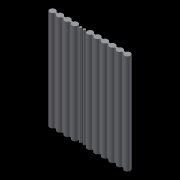
# Autodesk Inventor part: 3d_LM-Welding_Tooling - Wire Jacket
Saved by Autodesk Inventor 2018.3 (Build 223284000, 284)
## iProperties
Created: 2026-01-21
Part Number: 3d_LM-Welding_Tooling - Wire Jacket
Material: Genérico
Document SubType Name: Modeling
Designer: aca6
Density: 1 g/cm^3
Appearance: Valor por defecto
Author: aca6
Autodesk Inventor part; units mm, degrees
ref_plane "YZ Plane" through (0, 0, 0) normal (1, 0, 0) x (0, 1, 0)
ref_plane "XZ Plane" through (0, 0, 0) normal (0, 1, 0) x (-1, 0, 0)
ref_plane "XY Plane" through (0, 0, 0) normal (0, 0, 1) x (1, 0, 0)
sketch "Sketch1" plane through (0, 0, 0) normal (0, 0, 1) x (1, 0, 0)
  line L0 (25, -2) -> (24.25, -2) projected
  line L1 (25, 2) -> (25, -2) projected
  line L2 (24.25, 2) -> (25, 2) projected
  arc A0 (20.8229, 1.5) -> (24.25, 2) centre (22.5, 2) ccw projected
  line L3 (19.6771, 1.5) -> (20.8229, 1.5) projected
  arc A1 (16.3229, 1.5) -> (19.6771, 1.5) centre (18, 2) ccw projected
  line L4 (15.1771, 1.5) -> (16.3229, 1.5) projected
  arc A2 (11.8229, 1.5) -> (15.1771, 1.5) centre (13.5, 2) ccw projected
  line L5 (10.6771, 1.5) -> (11.8229, 1.5) projected
  arc A3 (7.3229, 1.5) -> (10.6771, 1.5) centre (9, 2) ccw projected
  line L6 (6.1771, 1.5) -> (7.3229, 1.5) projected
  arc A4 (2.8229, 1.5) -> (6.1771, 1.5) centre (4.5, 2) ccw projected
  line L7 (1.6771, 1.5) -> (2.8229, 1.5) projected
  arc A5 (-1.6771, 1.5) -> (1.6771, 1.5) centre (0, 2) ccw projected
  line L8 (-2.8229, 1.5) -> (-1.6771, 1.5) projected
  arc A6 (-6.1771, 1.5) -> (-2.8229, 1.5) centre (-4.5, 2) ccw projected
  line L9 (-7.3229, 1.5) -> (-6.1771, 1.5) projected
  arc A7 (-10.6771, 1.5) -> (-7.3229, 1.5) centre (-9, 2) ccw projected
  line L10 (-11.8229, 1.5) -> (-10.6771, 1.5) projected
  arc A8 (-15.1771, 1.5) -> (-11.8229, 1.5) centre (-13.5, 2) ccw projected
  line L11 (-16.3229, 1.5) -> (-15.1771, 1.5) projected
  arc A9 (-19.6771, 1.5) -> (-16.3229, 1.5) centre (-18, 2) ccw projected
  line L12 (-20.8229, 1.5) -> (-19.6771, 1.5) projected
  arc A10 (-24.25, 2) -> (-20.8229, 1.5) centre (-22.5, 2) ccw projected
  line L13 (-25, 2) -> (-24.25, 2) projected
  line L14 (-25, -2) -> (-25, 2) projected
  line L15 (-24.25, -2) -> (-25, -2) projected
  arc A11 (-20.8229, -1.5) -> (-24.25, -2) centre (-22.5, -2) ccw projected
  line L16 (-19.6771, -1.5) -> (-20.8229, -1.5) projected
  arc A12 (-16.3229, -1.5) -> (-19.6771, -1.5) centre (-18, -2) ccw projected
  line L17 (-15.1771, -1.5) -> (-16.3229, -1.5) projected
  arc A13 (-11.8229, -1.5) -> (-15.1771, -1.5) centre (-13.5, -2) ccw projected
  line L18 (-10.6771, -1.5) -> (-11.8229, -1.5) projected
  arc A14 (-7.3229, -1.5) -> (-10.6771, -1.5) centre (-9, -2) ccw projected
  line L19 (-6.1771, -1.5) -> (-7.3229, -1.5) projected
  arc A15 (-2.8229, -1.5) -> (-6.1771, -1.5) centre (-4.5, -2) ccw projected
  line L20 (-1.6771, -1.5) -> (-2.8229, -1.5) projected
  arc A16 (1.6771, -1.5) -> (-1.6771, -1.5) centre (0, -2) ccw projected
  line L21 (2.8229, -1.5) -> (1.6771, -1.5) projected
  arc A17 (6.1771, -1.5) -> (2.8229, -1.5) centre (4.5, -2) ccw projected
  line L22 (7.3229, -1.5) -> (6.1771, -1.5) projected
  arc A18 (10.6771, -1.5) -> (7.3229, -1.5) centre (9, -2) ccw projected
  line L23 (11.8229, -1.5) -> (10.6771, -1.5) projected
  arc A19 (15.1771, -1.5) -> (11.8229, -1.5) centre (13.5, -2) ccw projected
  line L24 (16.3229, -1.5) -> (15.1771, -1.5) projected
  arc A20 (19.6771, -1.5) -> (16.3229, -1.5) centre (18, -2) ccw projected
  line L25 (20.8229, -1.5) -> (19.6771, -1.5) projected
  arc A21 (24.25, -2) -> (20.8229, -1.5) centre (22.5, -2) ccw projected
  arc A22 (-8.7265, 4.65) -> (-8.4667, 4.5) centre (-8.4667, 4.8) ccw projected
  line L26 (-8.7265, 4.65) -> (-9.1941, 5.46) projected
  line L27 (-9.1941, 5.46) -> (-10.1962, 5.46) projected
  arc A23 (-12.1962, 5.46) -> (-10.1962, 5.46) centre (-11.1962, 5.46) ccw projected
  line L28 (-12.1962, 5.46) -> (-15.6962, 5.46) projected
  arc A24 (-17.6962, 5.46) -> (-15.6962, 5.46) centre (-16.6962, 5.46) ccw projected
  line L29 (-17.6962, 5.46) -> (-18.6983, 5.46) projected
  line L30 (-18.6983, 5.46) -> (-19.1659, 4.65) projected
  arc A25 (-19.4258, 4.5) -> (-19.1659, 4.65) centre (-19.4258, 4.8) ccw projected
  line L31 (-19.4258, 4.5) -> (-24, 4.5) projected
  arc A26 (-24, 4.5) -> (-25, 3.5) centre (-24, 3.5) ccw projected
  line L32 (-25, 3.5) -> (-25, 2) projected
  line L33 (-25, 2) -> (-24.25, 2) projected
  arc A27 (-20.8229, 2.5) -> (-24.25, 2) centre (-22.5, 2) ccw projected
  line L34 (-20.8229, 2.5) -> (-19.6771, 2.5) projected
  arc A28 (-16.3229, 2.5) -> (-19.6771, 2.5) centre (-18, 2) ccw projected
  line L35 (-16.3229, 2.5) -> (-15.1771, 2.5) projected
  arc A29 (-11.8229, 2.5) -> (-15.1771, 2.5) centre (-13.5, 2) ccw projected
  line L36 (-11.8229, 2.5) -> (-10.6771, 2.5) projected
  arc A30 (-7.3229, 2.5) -> (-10.6771, 2.5) centre (-9, 2) ccw projected
  line L37 (-7.3229, 2.5) -> (-6.1771, 2.5) projected
  arc A31 (-2.8229, 2.5) -> (-6.1771, 2.5) centre (-4.5, 2) ccw projected
  line L38 (-2.8229, 2.5) -> (-1.6771, 2.5) projected
  arc A32 (1.6771, 2.5) -> (-1.6771, 2.5) centre (0, 2) ccw projected
  line L39 (1.6771, 2.5) -> (2.8229, 2.5) projected
  arc A33 (6.1771, 2.5) -> (2.8229, 2.5) centre (4.5, 2) ccw projected
  line L40 (6.1771, 2.5) -> (7.3229, 2.5) projected
  arc A34 (10.6771, 2.5) -> (7.3229, 2.5) centre (9, 2) ccw projected
  line L41 (10.6771, 2.5) -> (11.8229, 2.5) projected
  arc A35 (15.1771, 2.5) -> (11.8229, 2.5) centre (13.5, 2) ccw projected
  line L42 (15.1771, 2.5) -> (16.3229, 2.5) projected
  arc A36 (19.6771, 2.5) -> (16.3229, 2.5) centre (18, 2) ccw projected
  line L43 (19.6771, 2.5) -> (20.8229, 2.5) projected
  arc A37 (24.25, 2) -> (20.8229, 2.5) centre (22.5, 2) ccw projected
  line L44 (24.25, 2) -> (25, 2) projected
  line L45 (25, 2) -> (25, 3.5) projected
  arc A38 (25, 3.5) -> (24, 4.5) centre (24, 3.5) ccw projected
  line L46 (24, 4.5) -> (-8.4667, 4.5) projected
  circle A39 centre (0, 2) radius 1.75
  circle A40 centre (-9, 2) radius 1.75
  circle A41 centre (-5.645, 2) radius 0.685
  circle A42 centre (-3.355, 2) radius 0.685
  line L47 (-4.5, 2) -> (-6.519, 2) construction
  line L48 (-7.3229, 1.5) -> (-6.1771, 1.5)
  line L49 (-2.8229, 1.5) -> (-1.6771, 1.5)
  line L50 (-1.6771, 2.5) -> (-2.8229, 2.5)
  circle A43 centre (-4.5, 2) radius 1.75
  line L51 (-6.1771, 2.5) -> (-7.3229, 2.5)
  point P0 (0, 0)
  dimension "d2" = 1.37
  dimension "d3" = 1.37
  dimension "d4" = 3.355
  dimension "d5" = 3.355
  constraints: 10 end point, 4 collinear, 3 centre point, 3 coincident, 2 horizontal, 2 horizontal alignment, 1 concentric, 6 other
  measures "d2" diameter of A41
  measures "d3" diameter of A42
  measures "d4" distance of A5.centre A42.centre
  measures "d5" distance of A7.centre A41.centre
extrude "Extrusion1" add sketch "Sketch1" along normal blind 60 contours A0 L3 A1 L4 A2 L5 A3 L6 A4 L7 A39 L39 A33 L40 A34 L41 A35 L42 A36 L43 A37 | A5 A39 A32 | L8 A43 A42 L38 A39 | L9 A40 L37 A43 A41 | A43 A42 | A42 A43 | A7 A40 A30 | A43 A41 | A41 A43 | L10 A8 L11 A9 L12 A10 A27 L34 A28 L35 A29 L36 A40
sketch "Sketch2" plane through (0, 0, 0) normal (0, 0, -1) x (-1, 0, 0)
  arc A0 (7.3229, 1.5) -> (10.6771, 1.5) centre (9, 2) ccw projected
  circle A1 centre (9, 2) radius 1.75
  arc A2 (10.6771, 2.5) -> (7.3229, 2.5) centre (9, 2) ccw projected
  line L0 (7.3229, 2.5) -> (6.1771, 2.5)
  arc A3 (6.2049, 2.3946) -> (6.2049, 1.6054) centre (5.645, 2) ccw projected
  circle A4 centre (5.645, 2) radius 0.685
  arc A5 (6.1771, 1.5) -> (6.2049, 1.6054) centre (4.5, 2) ccw projected
  line L1 (6.1771, 1.5) -> (6.2049, 1.6054)
  arc A6 (6.2049, 2.3946) -> (6.1771, 2.5) centre (4.5, 2) ccw projected
  line L2 (6.1771, 2.5) -> (6.2049, 2.3946)
  line L3 (6.1771, 1.5) -> (6.1771, 1.3136)
  line L4 (6.1771, 1.3136) -> (7.3763, 1.3471)
  line L5 (6.1771, 2.5) -> (6.1771, 2.7093)
  line L6 (6.1771, 2.7093) -> (7.416, 2.744)
  line L7 (4.5, 2) -> (4.5, 1.3471) construction
  arc A7 (-1.6771, 1.5) -> (1.6771, 1.5) centre (0, 2) ccw
  circle A8 centre (0, 2) radius 1.75
  arc A9 (1.6771, 2.5) -> (-1.6771, 2.5) centre (0, 2) ccw
  line L8 (1.6771, 2.5) -> (2.8229, 2.5)
  arc A10 (2.7951, 1.6054) -> (2.7951, 2.3946) centre (3.355, 2) ccw
  circle A11 centre (3.355, 2) radius 0.685
  arc A12 (2.7951, 1.6054) -> (2.8229, 1.5) centre (4.5, 2) ccw
  line L9 (2.8229, 1.5) -> (2.7951, 1.6054)
  arc A13 (2.8229, 2.5) -> (2.7951, 2.3946) centre (4.5, 2) ccw
  line L10 (2.8229, 2.5) -> (2.7951, 2.3946)
  line L11 (2.8229, 2.5) -> (2.8229, 2.7093)
  line L12 (2.8229, 2.7093) -> (1.584, 2.744)
  line L13 (2.8229, 1.5) -> (2.8229, 1.3136)
  line L14 (2.8229, 1.3136) -> (1.6237, 1.3471)
  point P0 (0, 0)
  dimension "d6" = 3.5
  dimension "d7" = 1.37
  constraints: 30 end point, 17 symmetric about line, 14 point on circle, 9 centre point, 4 coincident, 3 vertical, 1 collinear, 1 parallel, 7 other
  measures "d6" diameter of A1
  measures "d7" diameter of A4
extrude "Extrusion2" cut sketch "Sketch2" against normal blind 73.5 contours A0 L4 L3 A5 A4 A6 L0 A1 | A7 A8 L8 A13 A11 A12 L13 L14
body "Solid1"
